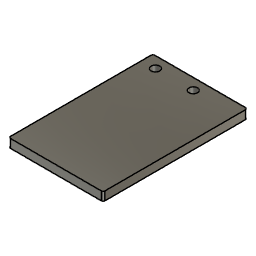
supporting part v14 (Autodesk Fusion 360 design; units mm, degrees)
Autodesk Fusion 360 part; units mm, degrees
sketch "草图1" plane through (0, 0, 0) normal (0, 0, 1) x (1, 0, 0)
  line L0 (-27.5, -48) -> (27.5, -48)
  line L1 (27.5, -48) -> (27.5, -132)
  line L2 (27.5, -132) -> (-27.5, -132)
  line L3 (-27.5, -48) -> (-27.5, -132)
  line L4 (0, 1.75) -> (0, 22.5)
  circle A0 centre (-19.5, -54.5) radius 2.5
  circle A1 centre (2.5, -54.5) radius 2.5
  dimension "d1" = 55
  dimension "d2" = 55
  dimension "d3" = 84
  dimension "d4" = 48
  dimension "d13" = 5
  dimension "d14" = 5
  dimension "d15" = 22
  dimension "d16" = 6.5
  dimension "d17" = 8
  constraint horizontal L0
  constraint perpendicular L0 L1
  constraint perpendicular L1 L2
  constraint symmetric L1.end L2.end L4
  constraint horizontal A0.centre A1.centre
  measures "d1" distance of L0.start L0.end
  measures "d2" distance of L1.end L2.end
  measures "d3" distance of L0.end L1.end
  measures "d4" vertical distance of origin L0.start
  measures "d13" diameter of A0
  measures "d14" diameter of A1
  measures "d15" horizontal distance of A0.centre A1.centre
  measures "d16" distance of L0 A0.centre
  measures "d17" distance of L3 A0.centre
extrude "拉伸1" add sketch "草图1" along normal blind 5
fillet "Fillet1" radius 1 4 edges at (-27.5, -48, 2.5) (27.5, -48, 2.5) (27.5, -132, 2.5) (-27.5, -132, 2.5)
equation "d14 = d13"
